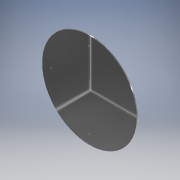
# Autodesk Inventor part: roundplate
Saved by Autodesk Inventor 2017 (Build 210142000, 142)
## iProperties
Created: 2016-10-09
Part Number: roundplate
Material: Aluminum 6061
Document SubType Name: Modeling
Designer: gus
Density: 2.7 g/cm^3
Appearance: Aluminum - Flat
Author: gus
Autodesk Inventor part; units mm, degrees
ref_plane "YZ Plane" through (0, 0, 0) normal (1, 0, 0) x (0, 1, 0)
ref_plane "XZ Plane" through (0, 0, 0) normal (0, 1, 0) x (-1, 0, 0)
ref_plane "XY Plane" through (0, 0, 0) normal (0, 0, 1) x (1, 0, 0)
sketch "Sketch1" plane through (0, 0, 0) normal (0, 0, 1) x (1, 0, 0)
  circle A0 centre (0, 0) radius 149.225
  circle A1 centre (0, 0) radius 120.2563 construction
  circle A2 centre (120.2563, 0) radius 2.5781
  circle A3 centre (0, 120.2563) radius 2.5781
  circle A4 centre (-120.2563, 0) radius 2.5781
  circle A5 centre (0, -120.2563) radius 2.5781
  line L0 (120.2563, 0) -> (0, 0) construction
  line L1 (0, 0) -> (0, 120.2563) construction
  line L2 (0, 0) -> (0, -120.2563) construction
  line L3 (0, 0) -> (-120.2563, 0) construction
  circle A6 centre (3.175, -146.05) radius 1.1557
  circle A7 centre (-3.175, -146.05) radius 1.1557
  line L4 (0, -120.2563) -> (0, -149.225) construction
  line L5 (3.175, -146.05) -> (0, -146.05) construction
  line L6 (0, -146.05) -> (-3.175, -146.05) construction
  dimension "d0" = 298.45
  dimension "d1" = 240.5126
  dimension "d2" = 5.1562
  dimension "d3" = 5.1562
  dimension "d4" = 5.1562
  dimension "d5" = 5.1562
  dimension "d8" = 2.3114
  dimension "d9" = 2.3114
  dimension "d10" = 146.05
  dimension "d11" = 3.175
  constraints: 14 end point, 7 centre point, 4 point on circle, 3 collinear, 3 perpendicular, 2 coincident, 2 point on line, 1 horizontal, 1 vertical alignment, 2 other
  measures "d1" diameter of A1
  measures "d2" diameter of A2
  measures "d3" diameter of A3
  measures "d4" diameter of A4
  measures "d5" diameter of A5
  measures "d8" diameter of A6
  measures "d9" diameter of A7
  measures "d10" distance from line of point (0, 0) L6
  measures "d11" distance of L5.end L6.end
extrude "Extrusion1" add sketch "Sketch1" along normal blind 3.175 contours A0 | A6 | A7
extrude "Extrusion2" cut sketch "Sketch1" along normal blind 3.175 contours A6 | A7
body "Solid1"
